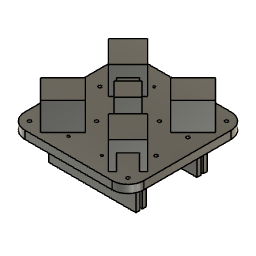
new_drone_base v5 (Autodesk Fusion 360 archive; units mm, degrees)
design "new_drone_base"
part number: Configuration 1
Autodesk Fusion 360 part; units mm, degrees
sketch "Sketch1" plane through (0, 0, 0) normal (0, 0, 1) x (1, 0, 0)
  line L0 (55, -75) -> (-55, -75)
  line L1 (-75, -55) -> (-75, 55)
  line L2 (-55, 75) -> (55, 75)
  line L3 (75, 55) -> (75, -55)
  line L4 (75, -75) -> (-75, 75) construction
  line L5 (-75, -75) -> (75, 75) construction
  line L6 (21, -54) -> (-21, 54) construction
  line L7 (-21, -54) -> (21, 54) construction
  line L8 (55.5, -20) -> (-55.5, 20) construction
  line L9 (-55.5, -20) -> (55.5, 20) construction
  line L10 (0, -17.6777) -> (-17.6777, 0)
  line L11 (-17.6777, 0) -> (0, 17.6777)
  line L12 (0, 17.6777) -> (17.6777, 0)
  line L13 (17.6777, 0) -> (0, -17.6777)
  line L14 (0, -17.6777) -> (0, 17.6777) construction
  line L15 (-17.6777, 0) -> (17.6777, 0) construction
  line L16 (0, 0) -> (-19.799, 19.799)
  line L17 (0, 0) -> (19.799, 19.799)
  line L18 (0, 0) -> (19.799, -19.799)
  line L19 (0, 0) -> (-19.799, -19.799)
  line L20 (-19.799, 19.799) -> (-26.8701, 26.8701)
  line L21 (0, 0) -> (0.539, 1.3859)
  line L22 (0, 0) -> (-0.539, 1.3859)
  line L23 (-17.6777, 0) -> (-27.6369, 9.9593)
  line L24 (0, 17.6777) -> (-11.2494, 28.9271)
  line L25 (19.799, 19.799) -> (26.8701, 26.8701)
  line L26 (-39.2444, 14.4957) -> (-67.5287, 42.78)
  line L27 (-14.4957, 39.2444) -> (-42.78, 67.5287)
  line L28 (-67.5287, 42.78) -> (-42.78, 67.5287)
  line L29 (-39.2444, 14.4957) -> (-14.4957, 39.2444)
  line L30 (39.2444, 14.4957) -> (67.5287, 42.78)
  line L31 (67.5287, 42.78) -> (42.78, 67.5287)
  line L32 (14.4957, 39.2444) -> (42.78, 67.5287)
  line L33 (39.2444, 14.4957) -> (14.4957, 39.2444)
  line L34 (-39.2444, -14.4957) -> (-67.5287, -42.78)
  line L35 (-67.5287, -42.78) -> (-42.78, -67.5287)
  line L36 (-14.4957, -39.2444) -> (-42.78, -67.5287)
  line L37 (-39.2444, -14.4957) -> (-14.4957, -39.2444)
  line L38 (39.2444, -14.4957) -> (67.5287, -42.78)
  line L39 (39.2444, -14.4957) -> (14.4957, -39.2444)
  line L40 (14.4957, -39.2444) -> (42.78, -67.5287)
  line L41 (67.5287, -42.78) -> (42.78, -67.5287)
  circle A0 centre (-55.5, 20) radius 2
  circle A1 centre (-55.5, -20) radius 2
  circle A2 centre (55.5, 20) radius 2
  circle A3 centre (55.5, -20) radius 2
  circle A4 centre (-21, 54) radius 1.5
  circle A5 centre (21, 54) radius 1.5
  circle A6 centre (-21, -54) radius 1.5
  circle A7 centre (21, -54) radius 1.5
  circle A8 centre (19.799, 19.799) radius 2
  circle A9 centre (-19.799, 19.799) radius 2
  circle A10 centre (-19.799, -19.799) radius 2
  circle A11 centre (19.799, -19.799) radius 2
  arc A12 (-55, 75) -> (-75, 55) centre (-55, 55) ccw
  arc A13 (75, 55) -> (55, 75) centre (55, 55) ccw
  arc A14 (-75, -55) -> (-55, -75) centre (-55, -55) ccw
  arc A15 (55, -75) -> (75, -55) centre (55, -55) ccw
  line L42 (-55, -55) -> (-62.0711, -62.0711)
  circle A16 centre (-62.0711, -62.0711) radius 2
  line L43 (-55, 55) -> (-62.0711, 62.0711)
  circle A17 centre (-62.0711, 62.0711) radius 2
  line L44 (55, 55) -> (62.0711, 62.0711)
  circle A18 centre (62.0711, 62.0711) radius 2
  line L45 (55, -55) -> (62.0711, -62.0711)
  circle A19 centre (62.0711, -62.0711) radius 2
  dimension "d1" = 150
  dimension "d2" = 150
  dimension "d3" = 42
  dimension "d4" = 108
  dimension "d5" = 111
  dimension "d6" = 40
  dimension "d7" = 25
  dimension "d8" = 25
  dimension "d9" = 28
  dimension "d10" = 28
  dimension "d11" = 28
  dimension "d12" = 28
  dimension "d15" = 10
  dimension "d21" = 17.5
  dimension "d22" = 17.5
  dimension "d23" = 40
  dimension "d24" = 40
  dimension "d25" = 4
  dimension "d26" = 4
  dimension "d27" = 4
  dimension "d28" = 4
  dimension "d29" = 3
  dimension "d30" = 3
  dimension "d31" = 3
  dimension "d32" = 3
  dimension "d33" = 4
  dimension "d34" = 4
  dimension "d35" = 4
  dimension "d36" = 4
  dimension "d43" = 20
  dimension "d44" = 20
  dimension "d45" = 20
  dimension "d46" = 20
  dimension "d68" = 10
  dimension "d69" = 4
  dimension "d70" = 10
  dimension "d71" = 4
  dimension "d72" = 10
  dimension "d73" = 4
  dimension "d74" = 10
  dimension "d75" = 4
  constraint horizontal L0
  constraint perpendicular L0 L1
  constraint parallel L0 L2
  constraint parallel L1 L3
  constraint coincident L4 L16.start
  constraint coincident L5 L16.start
  constraint coincident L16.start L17.start
  constraint coincident L6 L16.start
  constraint coincident L7 L16.start
  constraint coincident L8 L16.start
  constraint coincident L9 L16.start
  constraint perpendicular L10 L11
  constraint parallel L10 L12
  constraint parallel L11 L13
  constraint coincident L14 L16.start
  constraint coincident L15 L16.start
  constraint parallel L4 L16
  constraint parallel L5 L17
  constraint perpendicular L13 L18
  constraint perpendicular L10 L19
  constraint perpendicular L11 L23
  constraint perpendicular L11 L24
  constraint parallel L4 L20
  constraint coincident L7 L21.end
  constraint coincident L6 L22.end
  constraint coincident L8 L23.end
  constraint coincident L6 L24.end
  constraint parallel L5 L25
  constraint perpendicular L27 L29
  constraint coincident L8.end A0.centre
  constraint coincident L9.start A1.centre
  constraint coincident L9.end A2.centre
  constraint coincident L8.start A3.centre
  constraint coincident L6.end A4.centre
  constraint coincident L7.end A5.centre
  constraint coincident L7.start A6.centre
  constraint coincident L6.start A7.centre
  constraint coincident L17.end L25.start
  constraint coincident L16.end L20.start
  constraint coincident L19.end A10.centre
  constraint coincident L18.end A11.centre
  constraint coincident L4.end L2
  constraint coincident L4.end L1
  constraint tangent L2 A12
  constraint tangent L1 A12
  constraint coincident L5.end L2
  constraint coincident L5.end L3
  constraint tangent L2 A13
  constraint tangent L3 A13
  constraint coincident L5.start L1
  constraint coincident L5.start L0
  constraint tangent L1 A14
  constraint tangent L0 A14
  constraint coincident L4.start L0
  constraint coincident L4.start L3
  constraint tangent L0 A15
  constraint tangent L3 A15
  constraint coincident A14.centre L42.start
  constraint perpendicular L35 L42
  constraint coincident L42.end A16.centre
  constraint coincident A12.centre L43.start
  constraint perpendicular L28 L43
  constraint coincident L43.end A17.centre
  constraint coincident A13.centre L44.start
  constraint perpendicular L31 L44
  constraint coincident L44.end A18.centre
  constraint coincident A15.centre L45.start
  constraint perpendicular L41 L45
  constraint coincident L45.end A19.centre
  measures "d1" distance of L4.end L5.end
  measures "d2" distance of L5.start L4.end
  measures "d3" distance of L6.end L7.end
  measures "d4" distance of L7.start L6.end
  measures "d5" distance of L8.end L9.end
  measures "d6" distance of L9.start L8.end
  measures "d7" distance of L11.end L12.end
  measures "d8" distance of L10.end L11.end
  measures "d9" distance of L16.start L16.end
  measures "d10" distance of L16.start L17.end
  measures "d11" distance of L16.start L18.end
  measures "d12" distance of L16.start L19.end
  measures "d15" distance of L16.end L20.end
  measures "d21" distance of L20.end L27.start
  measures "d22" distance of L20.end L26.start
  measures "d23" distance of L26.start L26.end
  measures "d24" distance of L27.start L27.end
  measures "d25" diameter of A0
  measures "d26" diameter of A1
  measures "d27" diameter of A2
  measures "d28" diameter of A3
  measures "d29" diameter of A4
  measures "d30" diameter of A5
  measures "d31" diameter of A6
  measures "d32" diameter of A7
  measures "d33" diameter of A8
  measures "d34" diameter of A9
  measures "d35" diameter of A10
  measures "d36" diameter of A11
  measures "d43" radius of A12
  measures "d44" radius of A13
  measures "d45" radius of A14
  measures "d46" radius of A15
  measures "d68" distance of A14.centre L42.end
  measures "d69" diameter of A16
  measures "d70" distance of A12.centre L43.end
  measures "d71" diameter of A17
  measures "d72" distance of A13.centre L44.end
  measures "d73" diameter of A18
  measures "d74" distance of A15.centre L45.end
  measures "d75" diameter of A19
sketch "Sketch2" plane through (0, 0, 0) normal (0, 1, 0) x (1, 0, 0)
  line L0 (0, -12) -> (0, 12)
  constraint vertical L0
extrude "Extrude1" add sketch "Sketch1" against normal blind 10 contours L0 L1 L2 L3 A12 A13 A14 A15 | A16 | A17 | A18 | A19 makes body 1
extrude "Extrude2" add sketch "Sketch1" along normal blind 35 separate body contours L26 L27 L28 L29 | L30 L31 L32 L33 | L34 L35 L36 L37 | L38 L39 L40 L41 makes body 2 at (41.6014, 49.851, 0) makes body 3 at (40.4229, -32.1734, 0) makes body 4 at (-40.4229, 32.1734, 35) makes body 5 at (-23.9238, -48.6725, 11.6667)
extrude "Extrude3" add sketch "Sketch1" along normal blind 35 separate body contours L10 L13 L18 L19 | L10 L11 L16 L19 | L12 L13 L17 L18 | L11 L12 L16 L17 makes body 6
extrude "Extrude5" cut sketch "Sketch1" against normal blind 50 contours A16 | A17 | A18 | A19 bodies 1
sketch "Sketch5" plane through (-55.1543, -55.1543, 0) normal (-0.707107, -0.707107, 0) x (0.707107, -0.707107, 0)
  line L0 (-17.5, 0) -> (17.5, 0)
  line L1 (17.5, 0) -> (17.5, 35)
  line L2 (17.5, 35) -> (-17.5, 35)
  line L3 (-17.5, 35) -> (-17.5, 0)
  line L4 (0, 0) -> (0, 10.25)
  line L5 (10.25, 0) -> (-10.25, 0)
  line L6 (-10.25, 0) -> (-10.25, 20.5)
  line L7 (-10.25, 20.5) -> (10.25, 20.5)
  line L8 (10.25, 20.5) -> (10.25, 0)
  line L9 (10.25, 0) -> (-10.25, 20.5) construction
  line L10 (-10.25, 0) -> (10.25, 20.5) construction
  line L11 (-20, 0) -> (-19.5, 0)
  line L12 (-17.5, 2.5) -> (-17.5, 2)
  point P0 (0, 10.25)
  point P1 (-17.5, 0)
  dimension "d51" = 10.25
  dimension "d52" = 20.5
  dimension "d53" = 20.5
  dimension "d65" = 2
  constraint coincident L4.start origin
  constraint perpendicular L0 L4
  constraint horizontal L5
  constraint perpendicular L5 L6
  constraint parallel L5 L7
  constraint parallel L6 L8
  constraint coincident L9 P0
  constraint coincident L10 P0
  constraint coincident P0 L4.end
  constraint coincident L0.start L3.end
  constraint coincident L3 L12.end
  constraint coincident P1 L12
  constraint coincident P1 L11
  measures "d51" distance of L4.start P0
  measures "d52" distance of L6.end L7.end
  measures "d53" distance of L5.end L6.end
  measures "d65" distance of P1 L11.end
sketch "Sketch6" plane through (55.1543, -55.1543, 0) normal (0.707107, -0.707107, 0) x (0.707107, 0.707107, 0)
  line L0 (-17.5, 0) -> (17.5, 0)
  line L1 (17.5, 0) -> (17.5, 35)
  line L2 (17.5, 35) -> (-17.5, 35)
  line L3 (-17.5, 35) -> (-17.5, 0)
  line L4 (0, 0) -> (0, 10.25)
  line L5 (10.25, 0) -> (-10.25, 0)
  line L6 (-10.25, 0) -> (-10.25, 20.5)
  line L7 (-10.25, 20.5) -> (10.25, 20.5)
  line L8 (10.25, 20.5) -> (10.25, 0)
  line L9 (10.25, 0) -> (-10.25, 20.5) construction
  line L10 (-10.25, 0) -> (10.25, 20.5) construction
  point P0 (0, 10.25)
  dimension "d54" = 10.25
  dimension "d55" = 20.5
  dimension "d56" = 20.5
  constraint coincident L4.start origin
  constraint perpendicular L0 L4
  constraint horizontal L5
  constraint perpendicular L5 L6
  constraint parallel L5 L7
  constraint parallel L6 L8
  constraint coincident L9 P0
  constraint coincident L10 P0
  constraint coincident P0 L4.end
  measures "d54" distance of L4.start P0
  measures "d55" distance of L6.end L7.end
  measures "d56" distance of L5.end L6.end
sketch "Sketch7" plane through (55.1543, 55.1543, 0) normal (0.707107, 0.707107, 0) x (-0.707107, 0.707107, 0)
  line L0 (-17.5, 0) -> (17.5, 0)
  line L1 (17.5, 0) -> (17.5, 35)
  line L2 (17.5, 35) -> (-17.5, 35)
  line L3 (-17.5, 35) -> (-17.5, 0)
  line L4 (0, 0) -> (0, 10.25)
  line L5 (10.25, 0) -> (-10.25, 0)
  line L6 (-10.25, 0) -> (-10.25, 20.5)
  line L7 (-10.25, 20.5) -> (10.25, 20.5)
  line L8 (10.25, 20.5) -> (10.25, 0)
  line L9 (10.25, 0) -> (-10.25, 20.5) construction
  line L10 (-10.25, 0) -> (10.25, 20.5) construction
  point P0 (0, 10.25)
  dimension "d57" = 10.25
  dimension "d58" = 20.5
  dimension "d59" = 20.5
  constraint coincident L4.start origin
  constraint perpendicular L0 L4
  constraint horizontal L5
  constraint perpendicular L5 L6
  constraint parallel L5 L7
  constraint parallel L6 L8
  constraint coincident L9 P0
  constraint coincident L10 P0
  constraint coincident P0 L4.end
  measures "d57" distance of L4.start P0
  measures "d58" distance of L6.end L7.end
  measures "d59" distance of L5.end L6.end
sketch "Sketch8" plane through (-55.1543, 55.1543, 0) normal (-0.707107, 0.707107, 0) x (-0.707107, -0.707107, 0)
  line L0 (-17.5, 0) -> (17.5, 0)
  line L1 (17.5, 0) -> (17.5, 35)
  line L2 (17.5, 35) -> (-17.5, 35)
  line L3 (-17.5, 35) -> (-17.5, 0)
  line L4 (0, 0) -> (0, 10.25)
  line L5 (10.25, 0) -> (-10.25, 0)
  line L6 (-10.25, 0) -> (-10.25, 20.5)
  line L7 (-10.25, 20.5) -> (10.25, 20.5)
  line L8 (10.25, 20.5) -> (10.25, 0)
  line L9 (10.25, 0) -> (-10.25, 20.5) construction
  line L10 (-10.25, 0) -> (10.25, 20.5) construction
  point P0 (0, 10.25)
  dimension "d60" = 10.25
  dimension "d61" = 20.5
  dimension "d62" = 20.5
  constraint coincident L4.start origin
  constraint perpendicular L0 L4
  constraint horizontal L5
  constraint perpendicular L5 L6
  constraint parallel L5 L7
  constraint parallel L6 L8
  constraint coincident L9 P0
  constraint coincident L10 P0
  constraint coincident P0 L4.end
  measures "d60" distance of L4.start P0
  measures "d61" distance of L6.end L7.end
  measures "d62" distance of L5.end L6.end
move_face "OffsetFaces1" offset 10 4 faces at (41.6014, 49.851, 0) (40.4229, -32.1734, 0) (-40.4229, 32.1734, 0) (-32.1734, -40.4229, 0) on bodies 2 3 4 5
move_face "OffsetFaces2" offset 10 1 faces at (2.9463, -2.9463, 0) on bodies 6
sketch "Sketch9" plane through (0, 0, -10) normal (0, 0, -1) x (1, 0, 0)
  circle A0 centre (62.0711, 62.0711) radius 2
  circle A1 centre (-62.0711, -62.0711) radius 2
  circle A2 centre (-62.0711, 62.0711) radius 2
  circle A3 centre (62.0711, -62.0711) radius 2
  line L0 (-67.5287, 42.78) -> (-42.78, 67.5287)
  line L1 (-42.78, 67.5287) -> (-14.4957, 39.2444)
  line L2 (-14.4957, 39.2444) -> (-39.2444, 14.4957)
  line L3 (-39.2444, 14.4957) -> (-67.5287, 42.78)
  line L4 (-67.5287, -42.78) -> (-39.2444, -14.4957)
  line L5 (-39.2444, -14.4957) -> (-14.4957, -39.2444)
  line L6 (-14.4957, -39.2444) -> (-42.78, -67.5287)
  line L7 (-42.78, -67.5287) -> (-67.5287, -42.78)
  circle A4 centre (19.799, 19.799) radius 2
  circle A5 centre (-19.799, 19.799) radius 2
  circle A6 centre (19.799, -19.799) radius 2
  line L8 (17.6777, 0) -> (0, -17.6777)
  line L9 (0, -17.6777) -> (-17.6777, 0)
  line L10 (-17.6777, 0) -> (0, 17.6777)
  line L11 (0, 17.6777) -> (17.6777, 0)
  circle A7 centre (-19.799, -19.799) radius 2
  line L12 (67.5287, -42.78) -> (42.78, -67.5287)
  line L13 (42.78, -67.5287) -> (14.4957, -39.2444)
  line L14 (14.4957, -39.2444) -> (39.2444, -14.4957)
  line L15 (39.2444, -14.4957) -> (67.5287, -42.78)
  circle A8 centre (-55.5, 20) radius 2
  circle A9 centre (21, 54) radius 1.5
  circle A10 centre (-21, 54) radius 1.5
  circle A11 centre (21, -54) radius 1.5
  circle A12 centre (-21, -54) radius 1.5
  circle A13 centre (55.5, 20) radius 2
  circle A14 centre (-55.5, -20) radius 2
  circle A15 centre (55.5, -20) radius 2
  line L16 (39.2444, 14.4957) -> (14.4957, 39.2444)
  line L17 (14.4957, 39.2444) -> (42.78, 67.5287)
  line L18 (42.78, 67.5287) -> (67.5287, 42.78)
  line L19 (67.5287, 42.78) -> (39.2444, 14.4957)
  arc A16 (-55, 75) -> (-75, 55) centre (-55, 55) ccw
  line L20 (-75, 55) -> (-75, -55)
  arc A17 (-75, -55) -> (-55, -75) centre (-55, -55) ccw
  line L21 (-55, -75) -> (55, -75)
  arc A18 (55, -75) -> (75, -55) centre (55, -55) ccw
  line L22 (75, -55) -> (75, 55)
  arc A19 (75, 55) -> (55, 75) centre (55, 55) ccw
  line L23 (55, 75) -> (-55, 75)
  line L24 (55, -75) -> (55, -45)
  line L25 (-55, -75) -> (-55, -45)
  line L26 (-55, -45) -> (55, -45)
  line L27 (55, -45) -> (55, -40)
  line L28 (-55, -45) -> (-55, -40)
  line L29 (55, -40) -> (-55, -40)
  line L30 (0, 0) -> (100, 0)
  line L31 (55, -40) -> (55, -37)
  line L32 (-55, -40) -> (-55, -37)
  line L33 (55, -37) -> (-55, -37)
  line L34 (55, -37) -> (55, -32)
  line L35 (-55, -37) -> (-55, -32)
  line L36 (55, -32) -> (-55, -32)
  line L37 (55, 32) -> (-55, 32)
  line L38 (55, 37) -> (-55, 37)
  line L39 (55, 40) -> (-55, 40)
  line L40 (-55, 45) -> (55, 45)
  line L41 (55, 45) -> (55, 40)
  line L42 (55, 40) -> (55, 37)
  line L43 (55, 37) -> (55, 32)
  line L44 (-55, 37) -> (-55, 32)
  line L45 (-55, 40) -> (-55, 37)
  line L46 (-55, 45) -> (-55, 40)
  dimension "d82" = 5
  dimension "d83" = 5
  dimension "d84" = 100
  dimension "d85" = 3
  dimension "d86" = 3
  dimension "d87" = 5
  dimension "d88" = 5
  constraint coincident L21.end A18.start
  constraint perpendicular L21 L24
  constraint coincident A17.end L21.start
  constraint perpendicular L21 L25
  constraint perpendicular L24 L26
  constraint perpendicular L26 L27
  constraint perpendicular L26 L28
  constraint coincident L30.start origin
  constraint horizontal L30
  constraint perpendicular L29 L31
  constraint perpendicular L29 L32
  constraint perpendicular L33 L34
  constraint perpendicular L33 L35
  constraint symmetric L24.end L30 L40.end
  constraint symmetric L25.end L30 L40.start
  constraint symmetric L27.end L30 L39.start
  constraint symmetric L28.end L30 L39.end
  constraint symmetric L30 L31.end L38.start
  constraint symmetric L30 L32.end L38.end
  constraint symmetric L30 L34.end L37.start
  constraint symmetric L30 L35.end L37.end
  measures "d82" distance of L24.end L27.end
  measures "d83" distance of L25.end L28.end
  measures "d84" distance of L30.start L30.end
  measures "d85" distance of L27.end L31.end
  measures "d86" distance of L28.end L32.end
  measures "d87" distance of L31.end L34.end
  measures "d88" distance of L32.end L35.end
extrude "Extrude6" add sketch "Sketch9" along normal blind 40 contours L1 L17 L39 L40 | L1 L39 L40 L46 | L2 L37 L38 L44 | L2 L16 L37 L38 | L17 L39 L40 L41 | L16 L37 L38 L43 | L5 L14 L33 L36 | L5 L33 L35 L36 | L6 L26 L28 L29 | L14 L33 L34 L36 | L6 L13 L26 L29 | L13 L26 L27 L29 bodies 1 2 3 4 5
sketch "Sketch11" plane through (-55, 0, 0) normal (-1, 0, 0) x (0, -1, 0)
  line L0 (37, -10) -> (32, -10)
  line L1 (32, -10) -> (32, -50)
  line L2 (32, -50) -> (37, -50)
  line L3 (37, -50) -> (37, -10)
  arc A0 (32, -15) -> (27, -10) centre (27, -15) ccw
  line L4 (27, -10) -> (32, -10)
  arc A1 (50, -10) -> (45, -15) centre (50, -15) ccw
  line L5 (45, -10) -> (45, -15)
  line L6 (50, -10) -> (45, -10)
  arc A2 (-27, -10) -> (-32, -15) centre (-27, -15) ccw
  line L7 (-27, -10) -> (-32, -10)
  line L8 (-32, -10) -> (-32, -15)
  arc A3 (-45, -15) -> (-50, -10) centre (-50, -15) ccw
  line L9 (-45, -10) -> (-50, -10)
  line L10 (-45, -10) -> (-45, -15)
  point P0 (32, -10)
  point P1 (32, -10)
  point P2 (32, -10)
  point P3 (32, -10)
  point P4 (45, -10)
  point P5 (-32, -10)
  point P6 (-45, -10)
  dimension "d101" = 5
  dimension "d104" = 5
  dimension "d107" = 5
  dimension "d110" = 5
  constraint coincident P3 P1
  constraint coincident P3 P2
  constraint tangent A0 L4
  constraint coincident P4 L5.start
  constraint tangent A1 L5
  constraint tangent A1 L6
  constraint coincident P5 L7.end
  constraint tangent A2 L7
  constraint tangent A2 L8
  constraint coincident P6 L9.start
  constraint tangent A3 L9
  constraint tangent A3 L10
  measures "d101" radius of A0
  measures "d104" radius of A1
  measures "d107" radius of A2
  measures "d110" radius of A3
extrude "Extrude7" add sketch "Sketch11" against normal blind 110 contours L1 A0 L4 | A1 L5 L6 | A2 L7 L8 | A3 L9 L10 bodies 1
extrude "Extrude8" cut sketch "Sketch5" against normal blind 60 contours L0 L5 L6 L7 L8 bodies 1
extrude "Extrude9" cut sketch "Sketch6" against normal blind 60 contours L0 L5 L6 L7 L8 bodies 1
extrude "Extrude10" cut sketch "Sketch7" against normal blind 60 contours L0 L5 L6 L7 L8 bodies 1
extrude "Extrude11" cut sketch "Sketch8" against normal blind 60 contours L0 L5 L6 L7 L8 bodies 1
sketch "Sketch12" plane through (0, -45, 0) normal (0, -1, 0) x (1, 0, 0)
  line L0 (55, -15) -> (-55, -15)
  line L1 (-55, -15) -> (-55, -50)
  line L2 (-55, -50) -> (55, -50)
  line L3 (55, -50) -> (55, -15)
  line L4 (-55, -15) -> (-55, -30)
  circle A0 centre (-40, -30) radius 2
  circle A1 centre (40, -30) radius 2
  line L5 (-40, -30) -> (0, -30)
  circle A2 centre (0, -30) radius 2
  dimension "d121" = 15
  dimension "d122" = 15
  dimension "d124" = 4
  dimension "d125" = 4
  dimension "d128" = 40
  dimension "d129" = 4
  constraint coincident L0.end L1.start
  constraint coincident L1 L4.end
  constraint coincident A0.centre L5.start
  constraint horizontal L5
  constraint coincident L5.end A2.centre
  measures "d121" distance of L0.end L4.end
  measures "d122" distance of L4.end A0.centre
  measures "d124" diameter of A0
  measures "d125" diameter of A1
  measures "d128" distance of A0.centre L5.end
  measures "d129" diameter of A2
extrude "Extrude13" cut sketch "Sketch12" against normal blind 92 contours A0 | A1 | A2 bodies 1
